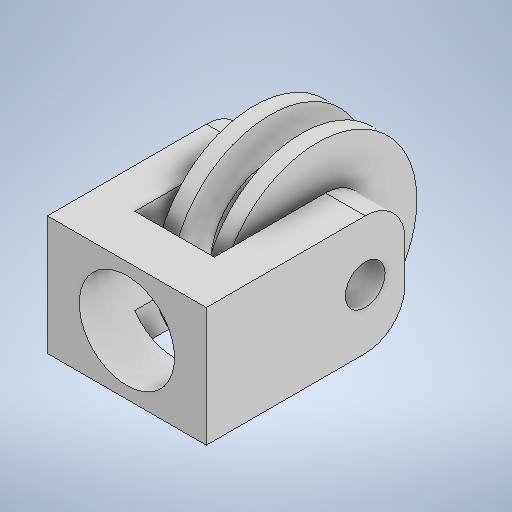
# Autodesk Inventor part: polea
Saved by Autodesk Inventor 2026 (Build 300175050, 175E)
## iProperties
Created: 2025-04-14
Part Number: polea
Material: Genérico
Document SubType Name: Modeling
Designer: piero
Density: 1 g/cm^3
Appearance: Valor por defecto
Author: piero
Autodesk Inventor part; units mm, degrees
sketch "Boceto1" plane through (0, 0, 0) normal (0, 0, 1) x (1, 0, 0)
  line L0 (0, 0) -> (20, 0)
  line L1 (20, 0) -> (20, 15)
  line L2 (20, 15) -> (0, 15)
  line L3 (0, 15) -> (0, 0)
  circle A0 centre (10, 7.5) radius 6
  dimension "d0" = 20
  dimension "d1" = 15
  dimension "d3" = 12
  constraints: 8 end point, 2 parallel, 1 centre point, 1 horizontal, 1 perpendicular
  measures "d0" distance of L2.end L1.end
  measures "d1" distance of L1.end L0.end
  measures "d3" diameter of A0
extrude "Extrusión1" add sketch "Boceto1" along normal blind 10
sketch "Boceto2" plane through (20, 0, 0) normal (1, 0, 0) x (0, 0, -1)
  line L0 (0, 0) -> (10, 0)
  line L1 (15, 5) -> (15, 10)
  line L2 (0, 0) -> (0, 15) projected
  line L3 (10, 15) -> (0, 15)
  arc A0 (15, 10) -> (10, 15) centre (10, 10) ccw
  arc A1 (10, 0) -> (15, 5) centre (10, 5) ccw
  circle A2 centre (10, 7.5) radius 2.5
  point P0 (15, 0)
  point P1 (15, 15)
  dimension "d6" = 15
  dimension "d7" = 15
  dimension "d9" = 5
  dimension "d10" = 5
  dimension "d11" = 5
  constraints: 6 end point, 4 point on circle, 4 point on line, 4 tangent, 3 centre point, 1 horizontal, 1 perpendicular
  measures "d6" distance of L0.start point (15, 0)
  measures "d7" distance of point (15, 0) point (15, 15)
  measures "d9" radius of A0
  measures "d10" radius of A1
  measures "d11" diameter of A2
extrude "Extrusión2" add sketch "Boceto2" against normal blind 5
sketch "Boceto3" plane through (0, 0, 0) normal (-1, 0, 0) x (0, 0, 1)
  line L0 (0, 15) -> (0, 10.8166) projected
  line L1 (0, 15) -> (-10, 15)
  line L2 (-15, 10) -> (-15, 5)
  line L3 (-10, 0) -> (0, 0)
  arc A0 (-10, 15) -> (-15, 10) centre (-10, 10) ccw
  arc A1 (-15, 5) -> (-10, 0) centre (-10, 5) ccw
  circle A2 centre (-10, 7.5) radius 2.5
  line L4 (0, 15) -> (0, 0)
  point P0 (-10, 15)
  point P1 (-15, 15)
  dimension "d14" = 15
  dimension "d15" = 5
  dimension "d16" = 5
  constraints: 8 end point, 4 point on circle, 4 tangent, 3 centre point, 2 perpendicular, 2 point on line, 1 equal radius, 1 horizontal, 1 vertical
  measures "d14" distance of L0.start point (-15, 15)
  measures "d15" radius of A0
  measures "d16" diameter of A2
extrude "Extrusión3" add sketch "Boceto3" against normal blind 5
ref_plane "Plano de trabajo1" through (14, 0, 10) normal (1, 0, 0) x (0, 0, -1)
ref_plane "Plano de trabajo3" through (6, 0, 10) normal (-1, 0, 0) x (0, 0, 1)
sketch "Boceto7" plane through (0, 0, 10) normal (0, -1, 0) x (1, 0, 0)
  line L0 (5, -10) -> (15, -10) projected
  line L1 (5, -10) -> (15, -10)
  line L2 (15, -10) -> (15, -6)
  line L3 (15, -6) -> (5, -6)
  line L4 (5, -6) -> (5, -10)
  point P0 (0, -10)
  dimension "d31" = 10
  dimension "d32" = 4
  constraints: 8 end point, 2 parallel, 1 horizontal, 1 perpendicular
  measures "d31" distance of L3.end L2.end
  measures "d32" distance of L2.end L1.end
extrude "Extrusión7" cut sketch "Boceto7" against normal blind 15
sketch "Boceto8" plane through (14, 0, 10) normal (1, 0, 0) x (0, 0, -1)
  circle A0 centre (20, 7.5) radius 2.5 projected
  circle A1 centre (20, 7.5) radius 12.5
  point P0 (10, 0)
  dimension "d35" = 25
  constraints: 1 centre point, 1 coincident
  measures "d35" diameter of A1
extrude "Extrusión8" add sketch "Boceto8" against normal blind 2
ref_plane "Plano de trabajo4" through (12, 7.5, -10) normal (1, 0, 0) x (0, 0, -1)
sketch "Boceto9" plane through (12, 7.5, -10) normal (1, 0, 0) x (0, 0, -1)
  circle A0 centre (0, 0) radius 7.5
  point P0 (-10, -7.5)
  dimension "d39" = 15
  constraints: 1 centre point
  measures "d39" diameter of A0
extrude "Extrusión9" add sketch "Boceto9" against normal blind 4
sketch "Boceto10" plane through (6, 0, 10) normal (-1, 0, 0) x (0, 0, 1)
  circle A0 centre (-20, 7.5) radius 2.5 projected
  circle A1 centre (-20, 7.5) radius 12.5
  circle A2 centre (-20, 7.5) radius 0.5
  circle A3 centre (-20, 7.5) radius 1.5
  point P0 (-10, 0)
  dimension "d42" = 25
  dimension "d47" = 1
  dimension "d48" = 3
  constraints: 3 centre point, 3 coincident
  measures "d42" diameter of A1
  measures "d47" diameter of A2
  measures "d48" diameter of A3
extrude "Extrusión10" add sketch "Boceto10" against normal blind 2 contours A1
sketch "Boceto11" plane through (12, 7.5, -10) normal (1, 0, 0) x (0, 0, -1)
  circle A0 centre (0, 0) radius 2.5
  point P0 (-10, -7.5)
  constraints: 1 centre point
extrude "Extrusión11" cut sketch "Boceto11" against normal blind 6
extrude "Extrusión12" add sketch "Boceto10" against normal blind 8 contours A2
